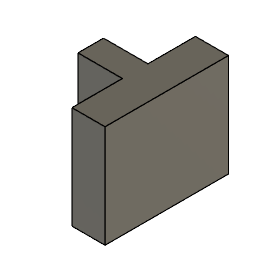
Button (Autodesk Fusion 360 design; units mm, degrees)
Autodesk Fusion 360 part; units mm, degrees
sketch "Sketch1" plane through (0, 0, 0) normal (0, 0, 1) x (1, 0, 0)
  line L0 (-1.05, 4.05) -> (1.15, 4.05)
  line L1 (1.15, 4.05) -> (1.15, -4.15)
  line L2 (1.15, -4.15) -> (-1.05, -4.15)
  line L3 (-1.05, 0.9) -> (-4, 0.9)
  line L4 (-4, 0.9) -> (-4, -0.8)
  line L5 (-4, -0.8) -> (-1.05, -0.8)
  line L6 (1.15, -0.9) -> (1.15, 0.9)
  line L7 (-1.05, -4.15) -> (-1.05, -0.8)
  line L8 (-1.05, 0.9) -> (-1.05, 4.05)
  dimension "d1" = 2.2
  dimension "d2" = 8.2
  dimension "d4" = 4.15
  dimension "d5" = 1.15
  dimension "d6" = 1.7
  dimension "d7" = 0.9
  dimension "d12" = 4
  constraint horizontal L0
  constraint vertical L1
  constraint horizontal L2
  constraint vertical L7
  constraint horizontal L3
  constraint vertical L4
  constraint horizontal L5
  constraint vertical L6
  constraint coincident L1 L6.end
  constraint collinear L7 L8
  measures "d1" distance of L0.start L0.end
  measures "d2" distance of L0.end L1.end
  measures "d4" distance of origin L2
  measures "d5" distance of origin L1
  measures "d6" distance of L3.end L4.end
  measures "d7" distance of origin L3
  measures "d12" distance of origin L4
extrude "Extrude1" add sketch "Sketch1" along normal blind 6.814
equation "d1 = 2.5 mm - 0.3 mm"
equation "d2 = 8.60 mm - 0.4 mm"
equation "d4 = ( 8.3 / 2 ) * 1 mm"
equation "d5 = ( 2.3 / 2 ) * 1 mm"
equation "d6 = 2 mm - 0.3 mm"
equation "d7 = ( 1.8 / 2 ) * 1 mm"
equation "d10 = 6.964 mm - 0.15 mm"
equation "d12 = 4.3 mm - 0.3 mm"
